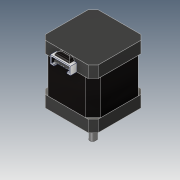
# Autodesk Inventor part: Nema_17
Saved by Autodesk Inventor 2021 (Build 250183000, 183)
## iProperties
Created: 2021-03-31
Part Number: Nema_17
Material: Ogólny
Document SubType Name: Modeling
Designer: mama
Density: 1 g/cm^3
Appearance: Gładki — czarny
Author: mama
Autodesk Inventor part; units mm, degrees
ref_plane "YZ Plane" through (0, 0, 0) normal (1, 0, 0) x (0, 1, 0)
ref_plane "XZ Plane" through (0, 0, 0) normal (0, 1, 0) x (-1, 0, 0)
ref_plane "XY Plane" through (0, 0, 0) normal (0, 0, 1) x (1, 0, 0)
sketch "Szkic1" plane through (0, 0, 0) normal (0, 1, 0) x (-1, 0, 0)
  line L0 (-21.15, 21.15) -> (21.15, 21.15)
  line L1 (21.15, 21.15) -> (21.15, -21.15)
  line L2 (21.15, -21.15) -> (-21.15, -21.15)
  line L3 (-21.15, -21.15) -> (-21.15, 21.15)
  line L4 (-21.15, 21.15) -> (21.15, -21.15) construction
  line L5 (21.15, 21.15) -> (-21.15, -21.15) construction
  point P0 (0, 0)
  dimension "d0" = 42.3
  dimension "d1" = 42.3
  constraints: 12 end point, 2 midpoint, 2 parallel, 1 horizontal, 1 perpendicular
  measures "d0" distance of L0.end L1.end
  measures "d1" distance of L1.end L2.end
extrude "Wyciągnięcie proste1" add sketch "Szkic1" along normal blind 9.4
chamfer "Faza1" distance 4 angle 45 4 edges at (21.15, 4.7, 21.15) (-21.15, 4.7, 21.15) (-21.15, 4.7, -21.15) (21.15, 4.7, -21.15)
sketch "Szkic2" plane through (0, 0, 0) normal (0, -1, 0) x (1, 0, 0)
  line L0 (21.15, -17.15) -> (17.15, -21.15) projected
  line L1 (21.15, -17.15) -> (21.15, 17.15) projected
  line L2 (17.15, 21.15) -> (21.15, 17.15) projected
  line L3 (17.15, 21.15) -> (-17.15, 21.15) projected
  line L4 (-21.15, 17.15) -> (-17.15, 21.15) projected
  line L5 (-21.15, 17.15) -> (-21.15, -17.15) projected
  line L6 (-17.15, -21.15) -> (-21.15, -17.15) projected
  line L7 (-17.15, -21.15) -> (17.15, -21.15) projected
  line L8 (21.15, -17.15) -> (21.15, 17.15) projected
  line L9 (21.15, 15) -> (21.15, -15)
  line L10 (17.15, -21.15) -> (-17.15, -21.15) projected
  line L11 (0, -21.15) -> (15, -21.15)
  line L12 (0, -21.15) -> (-15, -21.15)
  line L13 (-21.15, -17.15) -> (-21.15, 17.15) projected
  line L14 (-21.15, 0) -> (-21.15, -15)
  line L15 (-21.15, 0) -> (-21.15, 15)
  line L16 (-17.15, 21.15) -> (17.15, 21.15) projected
  line L17 (0, 21.15) -> (-15, 21.15)
  line L18 (0, 21.15) -> (15, 21.15)
  line L19 (21.15, 15) -> (15, 21.15)
  line L20 (21.15, -15) -> (15, -21.15)
  line L21 (-15, -21.15) -> (-21.15, -15)
  line L22 (-21.15, 15) -> (-15, 21.15)
  point P0 (0, 0)
  constraints: 22 end point, 8 point on line, 3 midpoint, 3 perpendicular
extrude "Wyciągnięcie proste2" add sketch "Szkic2" along normal blind 28.2 separate body contours L20 L7 L21 L5 L22 L3 L19 L1
sketch "Szkic3" plane through (0, -28.2, 0) normal (0, -1, 0) x (1, 0, 0)
  line L0 (21.15, -17.15) -> (17.15, -21.15) projected
  line L1 (21.15, -17.15) -> (21.15, 17.15) projected
  line L2 (17.15, 21.15) -> (21.15, 17.15) projected
  line L3 (17.15, 21.15) -> (-17.15, 21.15) projected
  line L4 (-21.15, 17.15) -> (-17.15, 21.15) projected
  line L5 (-21.15, 17.15) -> (-21.15, -17.15) projected
  line L6 (-17.15, -21.15) -> (-21.15, -17.15) projected
  line L7 (-17.15, -21.15) -> (17.15, -21.15) projected
  point P0 (0, 0)
extrude "Wyciągnięcie proste3" add sketch "Szkic3" along normal blind 9.4 separate body
sketch "Szkic4" plane through (0, -37.6, 0) normal (0, -1, 0) x (1, 0, 0)
  circle A0 centre (0, 0) radius 11.4
  dimension "d11" = 22.8
  constraints: 1 centre point, 1 coincident
  measures "d11" diameter of A0
extrude "Wyciągnięcie proste4" add sketch "Szkic4" along normal blind 2 bodies 3
sketch "Szkic5" plane through (0, -39.6, 0) normal (0, -1, 0) x (1, 0, 0)
  circle A0 centre (0, 0) radius 4
  dimension "d14" = 8
  constraints: 1 centre point, 1 coincident
  measures "d14" diameter of A0
extrude "Wyciągnięcie proste5" cut sketch "Szkic5" against normal blind 2 bodies 3
sketch "Szkic6" plane through (0, -37.6, 0) normal (0, -1, 0) x (1, 0, 0)
  circle A0 centre (0, 0) radius 2.75
  dimension "d17" = 5.5
  constraints: 1 centre point, 1 coincident
  measures "d17" diameter of A0
extrude "Wyciągnięcie proste6" cut sketch "Szkic6" against normal blind 2 bodies 3
sketch "Szkic7" plane through (0, -35.6, 0) normal (0, -1, 0) x (1, 0, 0)
  circle A0 centre (0, 0) radius 2.5
  dimension "d20" = 5
  constraints: 1 centre point, 1 coincident
  measures "d20" diameter of A0
extrude "Wyciągnięcie proste7" add sketch "Szkic7" along normal blind 25.5 separate body
sketch "Szkic8" plane through (0, -61.1, 0) normal (0, -1, 0) x (1, 0, 0)
  circle A0 centre (0, 0) radius 2.5 projected
  line L0 (2, 1.5) -> (2, -1.5)
  dimension "d23" = 4.5
  constraints: 2 end point, 2 point on circle, 1 vertical
extrude "Wyciągnięcie proste8" cut sketch "Szkic8" against normal blind 18 contours A0 L0 picked at (2.0912, -0.3466) bodies 4
sketch "Szkic9" plane through (0, -37.6, 0) normal (0, -1, 0) x (1, 0, 0)
  circle A0 centre (-15.5, -15.5) radius 1.5
  arc A1 (2, 1.5) -> (2, -1.5) centre (0, 0) ccw projected
  dimension "d26" = 3
  dimension "d27" = 15.5
  dimension "d28" = 15.5
  constraints: 1 centre point
  measures "d26" diameter of A0
  measures "d27" horizontal distance of A1.centre A0.centre
  measures "d28" horizontal distance of A1.centre A0.centre
extrude "Wyciągnięcie proste9" cut sketch "Szkic9" against normal blind 4 bodies 3
pattern_circular "Szyk kołowy1" count 4 over 360 about axis through (0, -35.6, 0) along (0, -1, 0) of "Wyciągnięcie proste9" bodies 3
thread "Gwint1" size "M3x0.5" class "6H" standard "ANSI Metric M Profile" full length
thread "Gwint2" size "M3x0.5" class "6H" standard "ANSI Metric M Profile" full length
thread "Gwint3" size "M3x0.5" class "6H" standard "ANSI Metric M Profile" full length
thread "Gwint4" size "M3x0.5" class "6H" standard "ANSI Metric M Profile" full length
chamfer "Faza2" distance 0.3 angle 45 4 edges at (-17, -37.6, -15.5) (-15.5, -37.6, 17) (15.5, -37.6, -17) (17, -37.6, 15.5)
sketch "Szkic10" plane through (0, 0, 0) normal (0, 1, 0) x (-1, 0, 0)
  line L0 (17.15, 21.15) -> (-17.15, 21.15) projected
  line L1 (0, 21.15) -> (-8.1, 21.15)
  line L2 (-8.1, 21.15) -> (-8.1, 26.15)
  line L3 (-8.1, 26.15) -> (8.1, 26.15)
  line L4 (8.1, 26.15) -> (8.1, 21.15)
  line L5 (0, 21.15) -> (8.1, 21.15)
  point P0 (0, 0)
  dimension "d45" = 8.1
  dimension "d46" = 5
  dimension "d47" = 16.2
  constraints: 10 end point, 2 perpendicular, 2 point on line, 1 collinear, 1 horizontal, 1 midpoint
  measures "d45" distance of L1.start L1.end
  measures "d46" distance of L1.end L2.end
  measures "d47" distance of L2.end L3.end
extrude "Wyciągnięcie proste10" add sketch "Szkic10" along normal blind 6.5 separate body
sketch "Szkic11" plane through (0, 9.4, 0) normal (0, 1, 0) x (1, 0, 0)
  line L0 (-17.15, -21.15) -> (17.15, -21.15) projected
  line L1 (0, -21.15) -> (6, -21.15)
  line L2 (6, -21.15) -> (6, -25)
  line L3 (6, -25) -> (-6, -25)
  line L4 (-6, -25) -> (-6, -21.15)
  line L5 (-6, -21.15) -> (0, -21.15)
  point P0 (0, 0)
  dimension "d50" = 3.85
  dimension "d51" = 12
  dimension "d52" = 11.15
  constraints: 10 end point, 3 perpendicular, 2 point on line, 1 midpoint
  measures "d50" distance of L1.end L2.end
  measures "d51" distance of L2.end L3.end
  measures "d52" distance from line of L0.end L2
extrude "Wyciągnięcie proste11" add sketch "Szkic11" against normal blind 2.9 separate body
fillet "Zaokrąglenie1" radius 2.9 3 edges at (6, 9.4, 23.075) (0, 9.4, 25) (-6, 9.4, 23.075)
sketch "Szkic12" plane through (-8.1, 0, 26.15) normal (0, 0, 1) x (1, 0, 0)
  line L0 (0, 0) -> (16.2, 0) projected
  line L1 (16.2, 0) -> (16.2, 6.5) projected
  line L2 (0, 6.5) -> (16.2, 6.5) projected
  line L3 (0, 0) -> (0, 6.5) projected
  line L4 (15.2, 1) -> (1, 1)
  line L5 (1, 1) -> (1, 5.5)
  line L6 (1, 5.5) -> (15.2, 5.5)
  line L7 (15.2, 5.5) -> (15.2, 1)
  point P0 (8.1, 0)
  dimension "d56" = 1
  constraints: 8 end point, 3 other
  measures "d56" distance between parallel lines of L0 L4
extrude "Wyciągnięcie proste12" cut sketch "Szkic12" against normal blind 4 contours L4 L5 L6 L7 bodies 5
sketch "Szkic13" plane through (-8.1, 0, 26.15) normal (0, 0, 1) x (1, 0, 0)
  line L0 (0, 0) -> (16.2, 0) projected
  line L1 (-6.9, 0) -> (23.1, 0) projected
  line L2 (15.2, 1) -> (1, 1) projected
  line L3 (13.2, 0) -> (3, 0)
  line L4 (3, 0) -> (3, 1)
  line L5 (3, 1) -> (13.2, 1)
  line L6 (13.2, 1) -> (13.2, 0)
  line L7 (15.2, 5.5) -> (15.2, 1) projected
  line L8 (1, 1) -> (1, 5.5) projected
  point P0 (8.1, 0)
  dimension "d59" = 2
  dimension "d60" = 2
  constraints: 8 end point, 2 parallel, 2 point on line, 1 horizontal, 1 perpendicular
  measures "d59" distance between parallel lines of L6 L7
  measures "d60" distance between parallel lines of L4 L8
extrude "Wyciągnięcie proste13" cut sketch "Szkic13" against normal blind 3 bodies 5
sketch "Szkic14" plane through (-8.1, 0, 22.15) normal (0, 0, 1) x (1, 0, 0)
  line L0 (15.2, 1) -> (13.2, 1) projected
  line L1 (15.2, 5.5) -> (15.2, 1) projected
  line L2 (15.2, 1) -> (1, 1) projected
  line L3 (15.2, 5.5) -> (15.2, 1) projected
  line L4 (1, 5.5) -> (15.2, 5.5) projected
  line L5 (1, 1) -> (1, 5.5) projected
  line L6 (15.2, 3.25) -> (1, 3.25)
  line L7 (13.6, 3.75) -> (12.6, 3.75)
  line L8 (12.6, 3.75) -> (12.6, 2.75)
  line L9 (12.6, 2.75) -> (13.6, 2.75)
  line L10 (13.6, 2.75) -> (13.6, 3.75)
  line L11 (13.6, 3.75) -> (12.6, 2.75) construction
  line L12 (12.6, 3.75) -> (13.6, 2.75) construction
  point P0 (8.1, 0)
  point P1 (13.1, 3.25)
  dimension "d63" = 1
  dimension "d64" = 2.1
  dimension "d65" = 1
  constraints: 14 end point, 4 midpoint, 2 parallel, 1 horizontal, 1 perpendicular, 1 point on line
  measures "d63" distance of L7.start L7.end
  measures "d64" distance of L6.start point (13.1, 3.25)
  measures "d65" distance of L7.end L8.end
extrude "Wyciągnięcie proste14" add sketch "Szkic14" along normal blind 3.5 separate body contours L10 L9 L8 L6 | L6 L8 L7 L10
pattern_linear "Szyk prostokątny1" count 6 spacing 2 along (-1, 0, 0) of "Wyciągnięcie proste14" bodies 7
